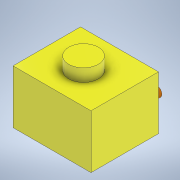
# Autodesk Inventor part: newcylinder1
Saved by Autodesk Inventor 2021 (Build 250183000, 183)
## iProperties
Created: 2021-07-24
Part Number: newcylinder1
Material: Generic
Document SubType Name: Modeling
Designer: Dell
Density: 1 g/cm^3
Appearance: Default
Author: Dell
Autodesk Inventor part; units mm, degrees
ref_plane "YZ Plane" through (0, 0, 0) normal (1, 0, 0) x (0, 1, 0)
ref_plane "XZ Plane" through (0, 0, 0) normal (0, 1, 0) x (-1, 0, 0)
ref_plane "XY Plane" through (0, 0, 0) normal (0, 0, 1) x (1, 0, 0)
sketch "Sketch1" plane through (0, 0, 0) normal (0, 0, 1) x (1, 0, 0)
  point P0 (0, 0)
sketch "Sketch2" plane through (0, 0, 0) normal (0, 0, 1) x (1, 0, 0)
  line L0 (-11.4108, 7.8651) -> (12.0555, 7.8651)
  line L1 (12.0555, 7.8651) -> (12.0555, -8.2519)
  line L2 (12.0555, -8.2519) -> (-11.4108, -8.2519)
  line L3 (-11.4108, -8.2519) -> (-11.4108, 7.8651)
  point P0 (0, 0)
  constraints: 8 end point, 2 parallel, 1 horizontal, 1 perpendicular
extrude "Extrusion1" add sketch "Sketch2" along normal blind 20.32
sketch "Sketch3" plane through (0, 0, 0) normal (0, 0, -1) x (-1, 0, 0)
  circle A0 centre (-8.9879, 0) radius 1.5322
  circle A1 centre (-4.3674, 0) radius 1.5722
  circle A2 centre (4.4307, 0) radius 1.5722
  circle A3 centre (8.7348, 0) radius 1.5671
  line L0 (-1.2026, 0.633) -> (1.2659, 0.633)
  line L1 (1.2659, 0.633) -> (1.2659, -1.1393)
  line L2 (1.2659, -1.1393) -> (-1.2026, -1.1393)
  line L3 (-1.2026, -1.1393) -> (-1.2026, 0.633)
  point P0 (0, 0)
  constraints: 8 end point, 4 centre point, 2 parallel, 1 horizontal, 1 perpendicular
extrude "Extrusion2" add sketch "Sketch3" along normal blind 2.54
sketch "Sketch4" plane through (-11.4108, 7.8651, 0) normal (0, 1, 0) x (1, 0, 0)
  circle A0 centre (11.7906, -10.8868) radius 4.4595
  point P0 (11.4108, 0)
  constraints: 1 centre point
extrude "Extrusion3" add sketch "Sketch4" along normal blind 3.81
body "Solid1"
